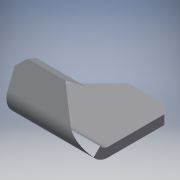
# Autodesk Inventor part: Part113
Saved by Autodesk Inventor 2016 (Build 200138000, 138)
## iProperties
Created: 2018-11-14
Part Number: Part113
Material: Generic
Document SubType Name: Sheet Metal
Designer: hovm
Density: 1 g/cm^3
Sheet Metal Rule: Default_mm
Appearance: Default
Author: hovm
Autodesk Inventor part; units mm, degrees
ref_plane "YZ Plane" through (0, 0, 0) normal (1, 0, 0) x (0, 1, 0)
ref_plane "XZ Plane" through (0, 0, 0) normal (0, 1, 0) x (-1, 0, 0)
ref_plane "XY Plane" through (0, 0, 0) normal (0, 0, 1) x (1, 0, 0)
sketch "Sketch1" plane through (0, 0, 0) normal (0, 0, 1) x (1, 0, 0)
  line L0 (-9, -10) -> (9, -10)
  line L1 (9, -10) -> (9, 10)
  line L2 (9, 10) -> (-9, 10)
  line L3 (-9, 10) -> (-9, -10)
  line L4 (-9, -10) -> (9, 10) construction
  line L5 (9, -10) -> (-9, 10) construction
  point P0 (0, 0)
  dimension "d0" = 18
  dimension "d1" = 20
  measures "d0" distance of L1.end L2.end
  measures "d1" distance of L0.end L1.end
extrude "Plate1" add sketch "Sketch1" along normal blind 2
sketch "Sketch2" plane through (9, -8.1451, -0.7479) normal (0, -0.9274452, 0.3739592) x (1, 0, 0)
  line L0 (-18, 0) -> (0, 0)
  line L1 (0, 0) -> (0, 12)
  line L2 (0, 12) -> (-18, 12)
  line L3 (-18, 12) -> (-18, 0)
  constraints: 6 end point, 1 horizontal, 1 perpendicular, 1 vertical
edge flange "Flange1" height 12 angle 111.96 thickness 2 bend radius 2 thickness toward (0, -0.9274452, 0.3739592) relief tear relief width 2 relief depth 1 edges at (0, -10, 2) wall of the first edge with corners at (-9, -8.1451, -0.7479) (9, -8.1451, -0.7479) (9, -3.6576, 10.3814) (-9, -3.6576, 10.3814)
bend "Bend1"
corner "Corner1"
chamfer "Corner Chamfer1" distance 2 angle 45 4 edges at (-9, 10, 1) (9, 10, 1) (-9, -4.585, 10.7554) (9, -4.585, 10.7554)
equation "\"d3\" = BendReliefWidth"
equation "\"d4\" = BendReliefDepth"
equation "\"d5\" = MinimumRemnant"
equation "\"d6\" = BendRadius"
equation "\"d9\" = BendRadius"
equation "\"d10\" = CornerReliefSize"
equation "\"d11\" = GapSize"
equation "\"d12\" = JacobiRadiusSize"
equation "\"BendRadius\" = Thickness"
equation "\"BendReliefWidth\" = Thickness"
equation "\"BendReliefDepth\" = 0.5 * Thickness"
equation "\"CornerReliefSize\" = 4 * Thickness"
equation "\"MinimumRemnant\" = 2 * Thickness"
equation "\"TransitionRadius\" = BendRadius"
equation "\"JacobiRadiusSize\" = BendRadius"
equation "\"GapSize\" = Thickness"
equation "\"d2\" = BendRadius"
equation "\"Thickness\" = 2"
body "Solid1"
